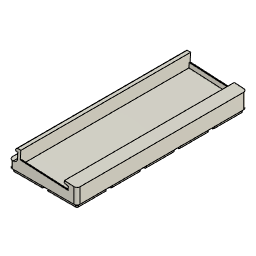
Gridfinity SMD Cassette Rail v10 (Autodesk Fusion 360 design; units mm, degrees)
Autodesk Fusion 360 part; units mm, degrees
ref_plane "WorkPlane1" through (0, 0, 7) normal (0, 0, 1) x (1, 0, 0) in component "Cassette Rail"
ref_plane "WorkPlane2" through (0, 0, 0.8) normal (0, 0, 1) x (1, 0, 0) in component "Cassette Rail"
ref_plane "WorkPlane3" through (0, 0, 2.6) normal (0, 0, 1) x (1, 0, 0) in component "Cassette Rail"
sketch "1U" plane through (0, 0, 7) normal (0, 0, 1) x (1, 0, 0) in component "Cassette Rail"
  line L0 (0, 0) -> (41.5, 0) construction
  line L1 (41.5, 0) -> (41.5, 41.5) construction
  line L2 (41.5, 41.5) -> (0, 41.5) construction
  line L3 (0, 41.5) -> (0, 0) construction
  line L4 (0, 37.75) -> (0, 3.75)
  arc A0 (0, 3.75) -> (3.75, 0) centre (3.75, 3.75) ccw
  line L5 (3.75, 0) -> (37.75, 0)
  arc A1 (37.75, 0) -> (41.5, 3.75) centre (37.75, 3.75) ccw
  line L6 (41.5, 3.75) -> (41.5, 37.75)
  arc A2 (41.5, 37.75) -> (37.75, 41.5) centre (37.75, 37.75) ccw
  line L7 (37.75, 41.5) -> (3.75, 41.5)
  arc A3 (3.75, 41.5) -> (0, 37.75) centre (3.75, 37.75) ccw
  line L8 (41.5, 41.5) -> (0, 0) construction
  dimension "d35" = 41.5
  dimension "d36" = 3.75
  constraint horizontal L0
  constraint vertical L1
  constraint horizontal L2
  constraint vertical L3
  constraint coincident L0.start L3.end
  constraint equal L1 L2
  constraint vertical L4
  constraint tangent L4 A0
  constraint tangent L5 A1
  constraint tangent L6 A2
  constraint tangent A2 L7
  constraint tangent L7 A3
  constraint coincident L4.start A3.end
  constraint horizontal L7
  constraint vertical L6
  constraint horizontal L5
  constraint tangent A0 L5
  constraint tangent L4 A3
  constraint tangent A1 L6
  constraint equal A0 A3
  constraint equal A2 A3
  constraint equal A1 A3
  constraint collinear L2 L7
  constraint collinear L3 L4
  constraint collinear L0 L5
  constraint collinear L1 L6
  measures "d35" distance of L0.start L0.end
  measures "d36" radius of A3
sketch "0.8" plane through (0, 0, 2.6) normal (0, 0, 1) x (1, 0, 0) in component "Cassette Rail"
  line L0 (2.15, 39.35) -> (39.35, 39.35) construction
  line L1 (39.35, 39.35) -> (39.35, 2.15) construction
  line L2 (39.35, 2.15) -> (2.15, 2.15) construction
  line L3 (2.15, 2.15) -> (2.15, 39.35) construction
  line L4 (2.15, 3.75) -> (2.15, 37.75)
  arc A0 (3.75, 39.35) -> (2.15, 37.75) centre (3.75, 37.75) ccw
  line L5 (3.75, 39.35) -> (37.75, 39.35)
  arc A1 (39.35, 37.75) -> (37.75, 39.35) centre (37.75, 37.75) ccw
  line L6 (39.35, 37.75) -> (39.35, 3.75)
  arc A2 (37.75, 2.15) -> (39.35, 3.75) centre (37.75, 3.75) ccw
  line L7 (37.75, 2.15) -> (3.75, 2.15)
  arc A3 (2.15, 3.75) -> (3.75, 2.15) centre (3.75, 3.75) ccw
  line L8 (0, 41.5) -> (0, 0) construction
  line L9 (2.15, 39.35) -> (39.35, 2.15) construction
  line L10 (41.5, 41.5) -> (0, 0) construction
  dimension "d37" = 2.15
  dimension "d38" = 1.6
  constraint horizontal L0
  constraint vertical L1
  constraint horizontal L2
  constraint vertical L3
  constraint vertical L4
  constraint tangent L4 A0
  constraint tangent A0 L5
  constraint tangent L5 A1
  constraint tangent A1 L6
  constraint tangent L6 A2
  constraint tangent A2 L7
  constraint tangent L7 A3
  constraint tangent L4 A3
  constraint horizontal L5
  constraint vertical L6
  constraint horizontal L7
  constraint equal A0 A1
  constraint equal A0 A3
  constraint equal A0 A2
  constraint collinear L0 L5
  constraint collinear L3 L4
  constraint collinear L2 L7
  constraint collinear L1 L6
  constraint equal L0 L3
  constraint midpoint L9 L10
  measures "d37" distance of L3 L8
  measures "d38" radius of A0
extrude "Extrude2" add sketch "0.8" against normal blind 1.8 makes body 1 in component "Cassette Rail"
extrude "Extrude3" add sketch "1U" against normal blind 2.25 separate body makes body 2 in component "Cassette Rail"
loft "Loft1" add section 1 face at (13.8333, 26.4167, 4.75) section 2 face at (26.4167, 15.6167, 2.6) on bodies 1 2 bodies 2 1 in component "Cassette Rail"
sketch "Sketch6" plane through (0, 0, 0) normal (0, 0, 1) x (1, 0, 0) in component "Cassette Rail"
  line L0 (2.95, 38.55) -> (38.55, 38.55) construction
  line L1 (38.55, 38.55) -> (38.55, 2.95) construction
  line L2 (38.55, 2.95) -> (2.95, 2.95) construction
  line L3 (2.95, 2.95) -> (2.95, 38.55) construction
  line L4 (2.95, 3.75) -> (2.95, 37.75)
  arc A0 (3.75, 38.55) -> (2.95, 37.75) centre (3.75, 37.75) ccw
  line L5 (3.75, 38.55) -> (37.75, 38.55)
  arc A1 (38.55, 37.75) -> (37.75, 38.55) centre (37.75, 37.75) ccw
  line L6 (38.55, 37.75) -> (38.55, 3.75)
  arc A2 (37.75, 2.95) -> (38.55, 3.75) centre (37.75, 3.75) ccw
  line L7 (37.75, 2.95) -> (3.75, 2.95)
  arc A3 (2.95, 3.75) -> (3.75, 2.95) centre (3.75, 3.75) ccw
  line L8 (2.15, 2.15) -> (2.15, 39.35)
  line L9 (2.95, 38.55) -> (38.55, 2.95) construction
  line L10 (41.5, 41.5) -> (0, 0) construction
  dimension "d43" = 0.8
  dimension "d44" = 0.8
  constraint horizontal L0
  constraint vertical L1
  constraint horizontal L2
  constraint vertical L3
  constraint tangent L4 A0
  constraint tangent L5 A1
  constraint tangent A1 L6
  constraint tangent L6 A2
  constraint tangent A2 L7
  constraint tangent L7 A3
  constraint coincident L4.start A3.start
  constraint tangent A0 L5
  constraint tangent L4 A3
  constraint equal A0 A3
  constraint equal A0 A1
  constraint equal A0 A2
  constraint collinear L0 L5
  constraint collinear L3 L4
  constraint collinear L2 L7
  constraint collinear L1 L6
  constraint midpoint L9 L10
  constraint equal L0 L1
  measures "d43" radius of A0
  measures "d44" distance of L3 L8
loft "Loft2" add profiles "Sketch6" section 1 face at (26.4167, 15.6167, 0.8) section 2 on bodies 2 bodies 2 in component "Cassette Rail"
sketch "Magnet Cutouts" plane through (0, 0, 0) normal (0, 0, -1) x (1, 0, 0) in component "Cassette Rail"
  spline S0 degree 3 poles (2.95, -37.75) (2.95, -30.1501) (2.95, -11.3499) (2.95, -3.75) (2.95, -3.6427) (2.9719, -3.5355) (3.0139, -3.4367) (3.0756, -3.2916) (3.1814, -3.1656) (3.3135, -3.0796) (3.4425, -2.9956) (3.5961, -2.95) (3.75, -2.95) (11.3499, -2.95) (30.1501, -2.95) (37.75, -2.95) (37.8573, -2.95) (37.9645, -2.9719) (38.0633, -3.0139) (38.2084, -3.0756) (38.3344, -3.1814) (38.4204, -3.3135) (38.5044, -3.4425) (38.55, -3.5961) (38.55, -3.75) (38.55, -11.3499) (38.55, -30.1501) (38.55, -37.75) (38.55, -37.8573) (38.5281, -37.9645) (38.4861, -38.0633) (38.4244, -38.2084) (38.3186, -38.3344) (38.1865, -38.4204) (38.0575, -38.5044) (37.9039, -38.55) (37.75, -38.55) (30.1501, -38.55) (11.3499, -38.55) (3.75, -38.55) (3.6427, -38.55) (3.5355, -38.5281) (3.4367, -38.4861) (3.2916, -38.4244) (3.1656, -38.3186) (3.0796, -38.1865) (2.9956, -38.0575) (2.95, -37.9039) (2.95, -37.75) knots 0 0 0 0 0.236941 0.236941 0.236941 0.240286 0.240286 0.240286 0.245202 0.245202 0.245202 0.25 0.25 0.25 0.486941 0.486941 0.486941 0.490286 0.490286 0.490286 0.495202 0.495202 0.495202 0.5 0.5 0.5 0.736941 0.736941 0.736941 0.740286 0.740286 0.740286 0.745202 0.745202 0.745202 0.75 0.75 0.75 0.986941 0.986941 0.986941 0.990286 0.990286 0.990286 0.995202 0.995202 0.995202 1 1 1 1 construction
  arc A0 (0, -37.75) -> (3.75, -41.5) centre (3.75, -37.75) ccw construction
  line L0 (0, -37.75) -> (0, -3.75) construction
  arc A1 (3.75, 0) -> (0, -3.75) centre (3.75, -3.75) ccw construction
  line L1 (3.75, 0) -> (37.75, 0) construction
  arc A2 (41.5, -3.75) -> (37.75, 0) centre (37.75, -3.75) ccw construction
  line L2 (41.5, -3.75) -> (41.5, -37.75) construction
  arc A3 (37.75, -41.5) -> (41.5, -37.75) centre (37.75, -37.75) ccw construction
  line L3 (37.75, -41.5) -> (3.75, -41.5) construction
  circle A4 centre (7.75, -7.75) radius 3.25
  line L4 (7.75, -7.75) -> (7.75, -2.95) construction
  line L5 (7.75, -7.75) -> (2.95, -7.75) construction
  line L6 (20.75, 0) -> (20.75, -41.5) construction
  line L7 (41.5, -20.75) -> (0, -20.75) construction
  circle A5 centre (33.75, -7.75) radius 3.25
  circle A6 centre (7.75, -33.75) radius 3.25
  circle A7 centre (33.75, -33.75) radius 3.25
  dimension "d108" = 6.5
  dimension "d109" = 4.8
  constraint coincident A4.centre L4.start
  constraint coincident S0 L4.end
  constraint vertical L4
  constraint coincident S0 L5.end
  constraint horizontal L5
  constraint equal L4 L5
  constraint midpoint L1 L6.start
  constraint midpoint L3 L6.end
  constraint midpoint L2 L7.start
  constraint midpoint L0 L7.end
  constraint symmetric A4 L6 A5
  constraint symmetric A4 L7 A6
  constraint symmetric L7 A5 A7
  measures "d108" diameter of A4
  measures "d109" distance of A4.centre L4.end
extrude "Extrude11" cut sketch "Magnet Cutouts" against normal blind 2.5 bodies 2 in component "Cassette Rail"
pattern_linear "R-Pattern1" count 2 spacing 42 along (1, 0, 0) count 5 spacing 42 along (0, 1, 0) of bodies 2 makes body 3 at (68.4167, 13.8333, 7) makes body 4 at (13.8333, 68.4167, 7) makes body 5 at (69.6667, 57.0833, 7) makes body 6 at (13.8333, 110.4167, 7) makes body 7 at (69.6667, 99.0833, 7) makes body 8 at (27.6667, 152.4167, 7) makes body 9 at (55.8333, 152.4167, 7) makes body 10 at (27.6667, 194.4167, 7) makes body 11 at (55.8333, 194.4167, 7) in component "Cassette Rail"
sketch "Base Plate Outside" plane through (0, 0, 7) normal (0, 0, 1) x (1, 0, 0) in component "Cassette Rail"
  line L0 (0, 0) -> (83.5, 0) construction
  line L1 (83.5, 0) -> (83.5, 209.5) construction
  line L2 (83.5, 209.5) -> (0, 209.5) construction
  line L3 (0, 209.5) -> (0, 0) construction
  line L4 (0, 3.75) -> (0, 205.75)
  arc A0 (3.75, 209.5) -> (0, 205.75) centre (3.75, 205.75) ccw
  line L5 (3.75, 209.5) -> (79.75, 209.5)
  arc A1 (83.5, 205.75) -> (79.75, 209.5) centre (79.75, 205.75) ccw
  line L6 (83.5, 205.75) -> (83.5, 3.75)
  arc A2 (79.75, 0) -> (83.5, 3.75) centre (79.75, 3.75) ccw
  line L7 (79.75, 0) -> (3.75, 0)
  arc A3 (0, 3.75) -> (3.75, 0) centre (3.75, 3.75) ccw
  dimension "d49" = 83.5
  dimension "d50" = 209.5
  dimension "d51" = 3.75
  constraint horizontal L0
  constraint vertical L1
  constraint horizontal L2
  constraint vertical L3
  constraint coincident L0.start L3.end
  constraint tangent L4 A0
  constraint tangent A0 L5
  constraint tangent L5 A1
  constraint tangent L6 A2
  constraint tangent L7 A3
  constraint tangent L4 A3
  constraint tangent A1 L6
  constraint tangent A2 L7
  constraint equal A0 A3
  constraint equal A0 A1
  constraint equal A0 A2
  constraint collinear L2 L5
  constraint collinear L1 L6
  constraint collinear L0 L7
  constraint collinear L3 L4
  measures "d49" distance of L1.end L2.end
  measures "d50" distance of L0.end L1.end
  measures "d51" radius of A0
extrude "Extrude4" add sketch "Base Plate Outside" along normal blind 40 and the other way up to surface (2.25 mm away) bodies 2 8 9 10 11 3 4 5 6 7 in component "Cassette Rail"
sketch "Rail Profile" plane through (0, 0, 0) normal (0, -1, 0) x (1, 0, 0) in component "Cassette Rail"
  line L0 (45.75, 4.75) -> (79.75, 4.75)
  line L1 (79.75, 4.75) -> (79.75, 47)
  line L2 (79.75, 47) -> (3.75, 47)
  line L3 (3.75, 47) -> (3.75, 4.75)
  line L4 (3.75, 4.75) -> (37.75, 4.75)
  line L5 (111.452, 8) -> (10.6173, 8) construction
  line L6 (111.452, 8) -> (0, 13.8409) construction
  line L7 (0, 13.8409) -> (9.8691, 13.3237)
  line L8 (10.5233, 25.8066) -> (7.827, 25.9479)
  line L9 (7.827, 25.9479) -> (7.9317, 27.9452)
  line L10 (7.9317, 27.9452) -> (10.0336, 29.8378)
  line L11 (10.0336, 29.8378) -> (14.2279, 29.6179)
  line L12 (14.2279, 29.6179) -> (13.3643, 13.1406)
  line L13 (72.2835, 10.0527) -> (72.8283, 20.4484)
  line L14 (72.8283, 20.4484) -> (67.8869, 21.6988)
  line L15 (67.8869, 21.6988) -> (68.023, 24.2952)
  line L16 (68.023, 24.2952) -> (83.5, 23.4841)
  line L17 (78.061, 24.7586) -> (77.2766, 9.7911) construction
  line L18 (83.5, 47) -> (0, 47)
  line L19 (10.5233, 25.8066) -> (9.8691, 13.3237)
  line L20 (10.0336, 29.8378) -> (9.9289, 27.8405) construction
  line L21 (7.9317, 27.9452) -> (9.9289, 27.8405) construction
  line L22 (13.3643, 13.1406) -> (72.2835, 10.0527)
  line L23 (13.6783, 19.1323) -> (72.5975, 16.0445)
  line L24 (12.5863, 84.2788) -> (9.1845, 19.3678) construction
  line L25 (9.1845, 19.3678) -> (72.0982, 16.0707) construction
  line L26 (72.0982, 16.0707) -> (75.5, 80.9816) construction
  line L27 (75.5, 80.9816) -> (12.5863, 84.2788) construction
  line L28 (44.0432, 82.6302) -> (40.6413, 17.7193) construction
  line L29 (83.5, 47) -> (83.5, 4.75) construction
  line L30 (83.5, 4.75) -> (83.5, 47)
  line L31 (83.5, 47) -> (83.5, 89.2064) construction
  line L32 (0, 4.75) -> (0, 47)
  line L33 (0, 47) -> (0, 4.75) construction
  line L34 (-21.0343, 88) -> (115.8166, 88) construction
  line L35 (1.75, 0) -> (22.5, 0) construction
  line L36 (37.75, 4.75) -> (45.75, 4.75)
  dimension "d67" = 3
  dimension "d68" = 2
  dimension "d69" = 4
  dimension "d70" = 6.2
  dimension "d71" = 3.5
  dimension "d72" = 59
  dimension "d73" = 5
  dimension "d74" = 111.6049
  dimension "d77" = 6
  dimension "d78" = 8
  dimension "d79" = 2.6
  dimension "d80" = 10.5
  dimension "d81" = 65
  dimension "d82" = 63
  dimension "d83" = 27
  dimension "d90" = 11.2
  dimension "d93" = 10
  dimension "d106" = 88
  dimension "d107" = 8
  constraint perpendicular L3 L5
  constraint coincident L6 L7.start
  constraint coincident L6 L7.end
  constraint perpendicular L6 L19
  constraint parallel L13 L17
  constraint parallel L13 L15
  constraint parallel L12 L13
  constraint parallel L12 L19
  constraint parallel L9 L12
  constraint perpendicular L11 L20
  constraint perpendicular L20 L21
  constraint equal L20 L21
  constraint perpendicular L13 L22
  constraint collinear L6 L22
  constraint coincident L13.end L14.start
  constraint coincident L12 L23.start
  constraint coincident L13 L23.end
  constraint perpendicular L13 L23
  constraint coincident L6 L17.end
  constraint perpendicular L24 L25
  constraint parallel L24 L26
  constraint parallel L25 L27
  constraint midpoint L27 L28.start
  constraint perpendicular L25 L28
  constraint perpendicular L23 L28
  constraint coincident L23 L28.end
  constraint collinear L23 L25
  constraint parallel L30 L31
  constraint horizontal L18
  constraint coincident L6.end L7.start
  constraint coincident L18.start L29.start
  constraint coincident L6.end L32
  constraint coincident L18.end L32.end
  constraint coincident L30 L16.end
  constraint horizontal L34
  measures "d67" angle of L5 L6
  measures "d68" distance of L10.end L20.end
  measures "d69" distance of L8 L11
  measures "d70" distance of L9 L12
  measures "d71" distance of L12 L19
  measures "d72" distance of L12 L13
  measures "d73" distance of L13 L17
  measures "d74" distance of L5.start L6.end
  measures "d77" distance of L22 L23
  measures "d78" distance of L16 L23
  measures "d79" distance of L14.end L15.end
  measures "d80" distance of L11 L23
  measures "d81" distance of L25.end L26.end
  measures "d82" distance of L24.start L26.end
  measures "d83" distance of L12 L28
  measures "d90" angle of L14 L16
  measures "d93" distance of L15 L17
  measures "d106" distance of L34 L35
  measures "d107" distance of L26.end L31
extrude "Extrude7" cut sketch "Rail Profile" against normal up to surface (209.5 mm away) contours L1 L2 L3 L7 L8 L9 L10 L11 L12 L13 L14 L15 L16 L18 L19 L23 | L1 L16 L18 L30 | L3 L7 L18 L32 | L12 L13 L22 L23 bodies 2 in component "Cassette Rail"
fillet "Fillet4" radius 5 1 edges at (9.8691, 104.75, 13.3237) on bodies 2 in component "Cassette Rail"
extrude "Extrude8" add sketch "Rail Profile" against normal blind 1.2 contours L12 L13 L22 L23 bodies 2 in component "Cassette Rail"
ref_plane "WorkPlane1" through (41.75, 104.75, 25.875) normal (0, 1, 0) x (1, 0, 0) in component "Cassette Rail"
mirror "Mirror1" about plane through (41.75, 104.75, 25.875) normal (0, 1, 0) of "Extrude8" in component "Cassette Rail"
ref_plane "WorkPlane2" through (0, 0, 19) normal (0, 0, 1) x (1, 0, 0) in component "Cassette Rail"
component "Cassette Rail" placed x (1, 0, 0) y (0, 1, 0) z (0, 0, 1) at (0, 0, 0)
equation "u = 7 mm"
equation "d4 = u"
equation "n_x = 2"
equation "n_y = 5"
equation "n_z = 3"
equation "d36 = ( 7.5 / 2 ) * 1 mm"
equation "d38 = ( 3.2 / 2 ) * 1 mm"
equation "d41 = -( u - ( 0.8 mm + 1.8 mm + 2.15 mm ) )"
equation "d43 = ( 1.6 / 2 ) * 1 mm"
equation "d45 = n_x"
equation "d46 = n_y"
equation "d49 = ( 42 * n_x - 0.5 ) * 1 mm"
equation "d50 = ( 42 * n_y - 0.5 ) * 1 mm"
equation "d51 = ( 7.5 / 2 ) * 1 mm"
equation "d77 = foam_thickness"
equation "foam_thickness = 6 mm"
named bodies: "GF SMD Casette Rail", "Body (1)", "Body (2)", "Body (3)", "Body (4)"
